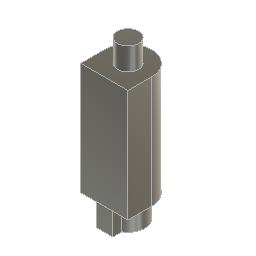
Post_Keyed_PostTop (Autodesk Fusion 360 design; units mm, degrees)
Autodesk Fusion 360 part; units mm, degrees
sketch "Sketch1" plane through (0, 0, 0) normal (0, 0, 1) x (1, 0, 0) in component "Post_Keyed_PostTop"
  circle A0 centre (0, 0) radius 1.5
  line L0 (-0.75, 0) -> (0.75, 0)
  line L1 (0.75, 0) -> (0.75, -2.1)
  line L2 (0.75, -2.1) -> (-0.75, -2.1)
  line L3 (-0.75, -2.1) -> (-0.75, 0)
  dimension "d11" = 3
  dimension "d25" = 1.5
  dimension "d26" = 2.1
  constraint coincident A0.centre origin
  constraint horizontal L0
  constraint vertical L1
  constraint horizontal L2
  constraint vertical L3
  constraint midpoint A0.centre L0
  measures "d11" diameter of A0
  measures "d25" distance of L0.start L0.end
  measures "d26" distance of L0.start L2.end
extrude "Extrude1" add sketch "Sketch1" against normal blind 2 contours A0 L0 L1 L3 | A0 L0 L1 L3 in component "Post_Keyed_PostTop"
sketch "Sketch2" plane through (0, 0, 0) normal (0, 0, 1) x (-1, 0, 0) in component "Post_Keyed_PostTop"
  circle A0 centre (0, 0) radius 1.5
  circle A1 centre (0, 0) radius 2.1
  dimension "d14" = 4.2
  constraint coincident A0.centre A1.centre
  measures "d14" diameter of A1
extrude "Extrude2" add sketch "Sketch2" along normal blind 10 contours A0 | A1 in component "Post_Keyed_PostTop"
sketch "Sketch3" plane through (0, 0, 10) normal (0, 0, 1) x (-1, 0, 0) in component "Post_Keyed_PostTop"
  circle A0 centre (0, 0) radius 2.1
  circle A1 centre (0, 0) radius 2.1
sketch "Sketch4" plane through (0, 0, 10) normal (0, 0, 1) x (-1, 0, 0) in component "Post_Keyed_PostTop"
  circle A0 centre (0, 0) radius 2.1
  line L0 (2.1, 0.0135) -> (-2.1, 0.0135)
  line L1 (-2.1, 0.0135) -> (-2.1, 2.1135)
  line L2 (-2.1, 2.1135) -> (2.1, 2.1135)
  line L3 (2.1, 2.1135) -> (2.1, 0.0135)
  dimension "d21" = 4.2
  dimension "d22" = 2.1
  constraint horizontal L0
  constraint vertical L1
  constraint horizontal L2
  constraint vertical L3
  constraint coincident A0 L0.start
  measures "d21" distance of L0.start L0.end
  measures "d22" distance of L0.start L2.end
extrude "Extrude3" add sketch "Sketch4" against normal up to surface (10 mm away) contours A0 L1 L2 L3 in component "Post_Keyed_PostTop"
extrude "Extrude4" add sketch "Sketch1" against normal up to surface (2 mm away) contours A0 L1 L2 L3 in component "Post_Keyed_PostTop"
sketch "Sketch5" plane through (0, 0, 10) normal (0, 0, 1) x (-1, 0, 0) in component "Post_Keyed_PostTop"
  arc A0 (-2.1, 0.0135) -> (2.1, 0.0135) centre (0, 0) ccw
  line L0 (2.1, 0.0135) -> (2.1, 2.1135)
  line L1 (2.1, 2.1135) -> (-2.1, 2.1135)
  line L2 (-2.1, 2.1135) -> (-2.1, 0.0135)
  circle A1 centre (0, 0) radius 0.95
  line L3 (-2.1, 0.0135) -> (-2.1, 0.0135)
  dimension "d32" = 1.9
  constraint coincident A0.centre A1.centre
  measures "d32" diameter of A1
extrude "Extrude5" add sketch "Sketch5" along normal blind 2 contours A1 in component "Post_Keyed_PostTop"
component "Post_Keyed_PostTop" placed x (1, 0, 0) y (0, 1, 0) z (0, 0, 1) at (0, 0, 0)
equation "Hole_Diameter = 3.2 mm"
equation "Print_Tolerance = 0.1 mm"
equation "Insert_Diameter = Hole_Diameter - Print_Tolerance"
equation "Flange_Overhang = 1 mm"
equation "Flange_Diameter = Hole_Diameter + Flange_Overhang"
equation "Post_Height = 10 mm"
equation "Bolt_Diameter = 2 mm"
equation "Bolt_Hole_Diameter = Bolt_Diameter - Print_Tolerance"
equation "Insert_Height = 2 mm"
equation "d11 = Insert_Diameter - Print_Tolerance"
equation "d12 = -Insert_Height"
equation "d14 = Flange_Diameter"
equation "d15 = Post_Height"
equation "Bolt_Hole_Depth = 5 mm"
equation "d21 = Flange_Diameter"
equation "d22 = Flange_Diameter / 2"
equation "d25 = ( Hole_Diameter / 2 ) - ( Print_Tolerance )"
equation "d26 = ( Flange_Diameter / 2 )"
equation "TopPost_Hole_Diameter = 2 mm"
equation "TopPost_Diameter = TopPost_Hole_Diameter - Print_Tolerance"
equation "TopPost_Height = 2 mm"
equation "d32 = TopPost_Diameter"
equation "d33 = TopPost_Height"
